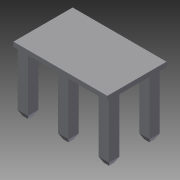
# Autodesk Inventor part: TMM-103-05-F-D_pins2
Saved by Autodesk Inventor 2014 SP2 (Build 180246200, 246)
## iProperties
Created: 2019-03-13
Part Number: TMM-103-05-F-D_pins2
Material: Generic
Catalog Web Link: www.cadenas.de
Description: TMM pins2-TMM Series
Vendor: SAMTEC
Document SubType Name: Modeling
Designer: psadmin
Manufacturer: SAMTEC
Mass: 0.00765058 g
Surface Area: 0.660321 cm^2
Volume: 0.00765058 cm^3
Density: 1 g/cm^3
Appearance: PSOLRGB-191-191-191
Category: PARTsolutions
Company: SAMTEC
Title: TMM-103-05-F-D_pins2
Author: Cadenas PARTsolutions
Comments: TMM Series
PSOL_IDENT_0: {$CADENAS_DATA\23d-libs\samtec\modelling\tmm\parts\tmm_pins2.prj},233 {VTYP=3D},{NB=TMM-103-05-F-D_p
PSOL_IDENT_1: ins2},{LINA=TMM-103-05-F-D_pins2},{NN=TMM pins2},{DATE=15.05.2015 12:28:13},{GEOMDATE=13.11.2014 09:
PSOL_IDENT_2: 06:00},{VERSION=},{LINEID=10},{WBVAR=POS,LS,PLOPT,ROW,TOPT,AOPT,RCOPT,POLOPT,KOPT,TROPT},{WBNUMERIC=
PSOL_IDENT_3: }  {NB=TMM-103-05-F-D_pins2},{LINA=TMM-103-05-F-D_pins2},{KT=DUMMY},{PN=TMM-103-05-F-D},{SERIES=TMM}
PSOL_IDENT_4: ,{POS=03},{LS=05},{LEADSTALG=},{PLOPT=F},{PLOPTALG= '-L','10micro\" (0,25 microm) Gold on contact, M
PSOL_IDENT_5: atte Tin on tail','-S','30micro\" (0,76 microm) Gold on contact, Matte Tin on tail' },{ROW=D},{ROWOP
PSOL_IDENT_6: TALG= 'S','S:Single row','D','D:Double Row','Q','Q:Quad Row' },{TOPT=},{TOPTALG= '','Straight','-SM'
PSOL_IDENT_7: ,'SM: Surface Mount' },{SH=160},{STACKERHALG=[120:323/5]},{TAILL=090},{TAILLALG='000','005','010','0
PSOL_IDENT_8: 15','020','025','030','035','040','045','050','055','060','065','070','075','080','085','090','095','
PSOL_IDENT_9: 100','105','110','115','120','125','130','135','140','145','150','155','160'},{AOPT=},{AOPTALG= '','
PSOL_IDENT_10: Not Available' },{RCOPT=},{RCOPTALG= '','Not Available' },{POLOPT=Not Selected},{POLARIZEALG='001','
PSOL_IDENT_11: 002','003','004','005','006'},{POLARIZEPN=},{KOPT=},{KOPTALG= '','Not Available' },{TROPT=},{TROPTAL
PSOL_IDENT_12: G= '','Not Available' },{L=0.23622},{W=0.1574},{OAL=0.323},{STACKERHMAX=323},{POLMAX='001','002','00
PSOL_IDENT_13: 3','004','005','006','007','008','009','010','011','012','013','014','015','016','017','018','019','
PSOL_IDENT_14: 020','021','022','023','024','025','026','027','028','029','030','031','032','033','034','035','036'
PSOL_IDENT_15: ,'037','038','039','040','041','042','043','044','045','046','047','048','049','050','051','052','05
PSOL_IDENT_16: 3','054','055','056','057','058','059','060','061','062','063','064','065','066','067','068','069','
PSOL_IDENT_17: 070','071','072','073','074','075','076','077','078','079','080','081','082','083','084','085','086'
PSOL_IDENT_18: ,'087','088','089','090','091','092','093','094','095','096','097','098','099','100','101','102','10
PSOL_IDENT_19: 3','104','105','106','107','108','109','110','111','112','113','114','115','116','117','118','119','
PSOL_IDENT_20: 120','121','122','123','124','125','126','127','128','129','130','131','132','133','134','135','136'
PSOL_IDENT_21: ,'137','138','139','140','141','142','143','144','145','146','147','148','149','150','151','152','15
PSOL_IDENT_22: 3','154','155','156','157','158','159','160','161','162','163','164','165','166','167','168','169','
PSOL_IDENT_23: 170','171','172','173','174','175','176','177','178','179','180','181','182','183','184','185','186'
PSOL_IDENT_24: ,'187','188','189','190','191','192','193','194','195','196','197','198','199','200','201','202','20
PSOL_IDENT_25: 3','204','205','206','207','208','209','210','211','212','213','214','215','216','217','218','219','
PSOL_IDENT_26: 220','221','222','223','224','225','226','227','228','229','230','231','232','233','234','235','236'
PSOL_IDENT_27: ,'237','238','239','240','241','242','243','244','245','246','247','248','249','250','251','252','25
PSOL_IDENT_28: 3','254','255','256','257','258','259','260','261','262','263','264','265','266','267','268','269','
PSOL_IDENT_29: 270','271','272','273','274','275','276','277','278','279','280','281','282','283','284','285','286'
PSOL_IDENT_30: ,'287','288','289','290','291','292','293','294','295','296','297','298','299','300'},{TEST2='001','
PSOL_IDENT_31: 002','003','004','005','006'},{TRUNC=6},{MIN=0.163},{PINSNUM=3},{POLLR=0},{TAILLMAX=163},{TAILLRANGE='
PSOL_IDENT_32: 000','005','010','015','020','025','030','035','040','045','050','055','060','065','070','075','080'
PSOL_IDENT_33: ,'085','090','095','100','105','110','115','120','125','130','135','140','145','150','155','160','16
PSOL_IDENT_34: 5','170','175','180','185','190','195','200','205','210','215','220','225','230','235','240','245','
PSOL_IDENT_35: 250','255','260','265','270','275','280','285','290','295','300','305','310','315','320','325','330'
PSOL_IDENT_36: ,'335','340','345','350','355','360','365','370','375','380','385','390','395','400','405','410','41
PSOL_IDENT_37: 5','420','425','430','435','440','445','450','455','460','465','470','475','480','485','490','495','
PSOL_IDENT_38: 500','505','510','515','520','525','530','535','540','545','550','555','560','565','570','575','580'
PSOL_IDENT_39: ,'585','590','595','600','605','610','615','620','625','630','635','640','645','650','655','660','66
PSOL_IDENT_40: 5','670','675','680','685','690','695','700','705','710','715','720','725','730','735','740','745','
PSOL_IDENT_41: 750','755','760','765','770','775','780','785','790','795','800','805','810','815','820','825','830'
PSOL_IDENT_42: ,'835','840','845','850','855','860','865','870','875','880','885','890','895','900','905','910','91
PSOL_IDENT_43: 5','920','925','930','935','940','945','950','955','960','965','970','975','980','985','990','995'},
PSOL_IDENT_44: {TAILLTRUNC=33},{TAILLNUM=0.09},{ROWNO=2},{POLPLANEPOS=0},{POLPINPOS=0},{TOPCUT=0.198},{COLOR=0.75,0
PSOL_IDENT_45: .75,0.75,0.00}
NN: TMM pins2
NT: TMM Series
NB: TMM-103-05-F-D_pins2
NBSYN: $PN._pins2
LINA: TMM-103-05-F-D_pins2
SERIES: TMM
POS: 03
LS: 05
PLOPT: -F: 3u" Selective Gold on Contact, Matte Tin on Tail
ROW: D:Double Row
TOPT: Straight
SH: 160
AOPT: Not Available
RCOPT: Not Available
POLOPT: Not Selected
KOPT: Not Available
TROPT: Not Available
POLMAX: '001','002','003','004','005','006','007','008','009','010','011','012','013','014','015','016','017','018','019','020','021','022','023','024','025','026','027','028','029','030','031','032','033','034','035','036','037','038','039','040','041','042','043','044','045','046','047','048','049','050','051','052','053','054','055','056','057','058','059','060','061','062','063','064','065','066','067','068','069','070','071','072','073','074','075','076','077','078','079','080','081','082','083','084','085','086','087','088','089','090','091','092','093','094','095','096','097','098','099','100','101','102','103','104','105','106','107','108','109','110','111','112','113','114','115','116','117','118','119','120','121','122','123','124','125','126','127','128','129','130','131','132','133','134','135','136','137','138','139','140','141','142','143','144','145','146','147','148','149','150','151','152','153','154','155','156','157','158','159','160','161','162','163','164','165','166','167','168','169','170','171','172','173','174','175','176','177','178','179','180','181','182','183','184','185','186','187','188','189','190','191','192','193','194','195','196','197','198','199','200','201','202','203','204','205','206','207','208','209','210','211','212','213','214','215','216','217','218','219','220','221','222','223','224','225','226','227','228','229','230','231','232','233','234','235','236','237','238','239','240','241','242','243','244','245','246','247','248','249','250','251','252','253','254','255','256','257','258','259','260','261','262','263','264','265','266','267','268','269','270','271','272','273','274','275','276','277','278','279','280','281','282','283','284','285','286','287','288','289','290','291','292','293','294','295','296','297','298','299','300'
TAILLRANGE: '000','005','010','015','020','025','030','035','040','045','050','055','060','065','070','075','080','085','090','095','100','105','110','115','120','125','130','135','140','145','150','155','160','165','170','175','180','185','190','195','200','205','210','215','220','225','230','235','240','245','250','255','260','265','270','275','280','285','290','295','300','305','310','315','320','325','330','335','340','345','350','355','360','365','370','375','380','385','390','395','400','405','410','415','420','425','430','435','440','445','450','455','460','465','470','475','480','485','490','495','500','505','510','515','520','525','530','535','540','545','550','555','560','565','570','575','580','585','590','595','600','605','610','615','620','625','630','635','640','645','650','655','660','665','670','675','680','685','690','695','700','705','710','715','720','725','730','735','740','745','750','755','760','765','770','775','780','785','790','795','800','805','810','815','820','825','830','835','840','845','850','855','860','865','870','875','880','885','890','895','900','905','910','915','920','925','930','935','940','945','950','955','960','965','970','975','980','985','990','995'
SUPPLIER: SAMTEC
ARTICLENO: TMM-103-05-F-D_pins2
BOMINFO: TMM-103-05-F-D_pins2
CREATOR: CADENAS GmbH
Autodesk Inventor part; units mm, degrees
ref_plane "YZ Plane" through (0, 0, 0) normal (1, 0, 0) x (0, 1, 0)
ref_plane "XZ Plane" through (0, 0, 0) normal (0, 1, 0) x (-1, 0, 0)
ref_plane "XY Plane" through (0, 0, 0) normal (0, 0, 1) x (1, 0, 0)
sketch "Sketch_2" plane through (-2.254, 0, 0) normal (1, 0, 0) x (0, 0, -1)
  line L0 (-1.4605, 0.762) -> (-1.254, 0.762)
  line L1 (-1.254, 0.762) -> (-1.254, -2.032)
  line L2 (-1.254, -2.032) -> (-1.127, -2.286)
  line L3 (-1.127, -2.286) -> (-0.873, -2.286)
  line L4 (-0.873, -2.286) -> (-0.746, -2.032)
  line L5 (-0.746, -2.032) -> (-0.746, 0.762)
  line L6 (-0.746, 0.762) -> (0.746, 0.762)
  line L7 (0.746, 0.762) -> (0.746, -2.032)
  line L8 (0.746, -2.032) -> (0.873, -2.286)
  line L9 (0.873, -2.286) -> (1.127, -2.286)
  line L10 (1.127, -2.286) -> (1.254, -2.032)
  line L11 (1.254, -2.032) -> (1.254, 0.762)
  line L12 (1.254, 0.762) -> (1.4605, 0.762)
  line L13 (1.4605, 0.762) -> (1.4605, 0.9906)
  line L14 (1.4605, 0.9906) -> (-1.4605, 0.9906)
  line L15 (-1.4605, 0.9906) -> (-1.4605, 0.762)
  constraints: 32 end point
extrude "Extrusion1" add sketch "Sketch_2" along normal blind 4.635
sketch "Sketch_1" plane through (0, 0, 0) normal (0, 0, 1) x (1, 0, 0)
  line L0 (-109.4334, 38.1) -> (-109.4334, -38.1)
  line L1 (-109.4334, -38.1) -> (56.7986, -38.1)
  line L2 (56.7986, -38.1) -> (56.7986, 38.1)
  line L3 (56.7986, 38.1) -> (-109.4334, 38.1)
  line L4 (-100.4603, 0.762) -> (-100.2538, 0.762)
  line L5 (-100.2538, 0.762) -> (-100.2538, -2.032)
  line L6 (-100.2538, -2.032) -> (-100.1268, -2.286)
  line L7 (-100.1268, -2.286) -> (-99.8728, -2.286)
  line L8 (-99.8728, -2.286) -> (-99.7458, -2.032)
  line L9 (-99.7458, -2.032) -> (-99.7458, 0.762)
  line L10 (-99.7458, 0.762) -> (-98.2538, 0.762)
  line L11 (-98.2538, 0.762) -> (-98.2538, -2.032)
  line L12 (-98.2538, -2.032) -> (-98.1268, -2.286)
  line L13 (-98.1268, -2.286) -> (-97.8728, -2.286)
  line L14 (-97.8728, -2.286) -> (-97.7458, -2.032)
  line L15 (-97.7458, -2.032) -> (-97.7458, 0.762)
  line L16 (-97.7458, 0.762) -> (-96.2538, 0.762)
  line L17 (-96.2538, 0.762) -> (-96.2538, -2.032)
  line L18 (-96.2538, -2.032) -> (-96.1268, -2.286)
  line L19 (-96.1268, -2.286) -> (-95.8728, -2.286)
  line L20 (-95.8728, -2.286) -> (-95.7458, -2.032)
  line L21 (-95.7458, -2.032) -> (-95.7458, 0.762)
  line L22 (-95.7458, 0.762) -> (-94.2538, 0.762)
  line L23 (-94.2538, 0.762) -> (-94.2538, -2.032)
  line L24 (-94.2538, -2.032) -> (-94.1268, -2.286)
  line L25 (-94.1268, -2.286) -> (-93.8728, -2.286)
  line L26 (-93.8728, -2.286) -> (-93.7458, -2.032)
  line L27 (-93.7458, -2.032) -> (-93.7458, 0.762)
  line L28 (-93.7458, 0.762) -> (-92.2538, 0.762)
  line L29 (-92.2538, 0.762) -> (-92.2538, -2.032)
  line L30 (-92.2538, -2.032) -> (-92.1268, -2.286)
  line L31 (-92.1268, -2.286) -> (-91.8728, -2.286)
  line L32 (-91.8728, -2.286) -> (-91.7458, -2.032)
  line L33 (-91.7458, -2.032) -> (-91.7458, 0.762)
  line L34 (-91.7458, 0.762) -> (-90.2538, 0.762)
  line L35 (-90.2538, 0.762) -> (-90.2538, -2.032)
  line L36 (-90.2538, -2.032) -> (-90.1268, -2.286)
  line L37 (-90.1268, -2.286) -> (-89.8728, -2.286)
  line L38 (-89.8728, -2.286) -> (-89.7458, -2.032)
  line L39 (-89.7458, -2.032) -> (-89.7458, 0.762)
  line L40 (-89.7458, 0.762) -> (-88.2538, 0.762)
  line L41 (-88.2538, 0.762) -> (-88.2538, -2.032)
  line L42 (-88.2538, -2.032) -> (-88.1268, -2.286)
  line L43 (-88.1268, -2.286) -> (-87.8728, -2.286)
  line L44 (-87.8728, -2.286) -> (-87.7458, -2.032)
  line L45 (-87.7458, -2.032) -> (-87.7458, 0.762)
  line L46 (-87.7458, 0.762) -> (-86.2538, 0.762)
  line L47 (-86.2538, 0.762) -> (-86.2538, -2.032)
  line L48 (-86.2538, -2.032) -> (-86.1268, -2.286)
  line L49 (-86.1268, -2.286) -> (-85.8728, -2.286)
  line L50 (-85.8728, -2.286) -> (-85.7458, -2.032)
  line L51 (-85.7458, -2.032) -> (-85.7458, 0.762)
  line L52 (-85.7458, 0.762) -> (-84.2538, 0.762)
  line L53 (-84.2538, 0.762) -> (-84.2538, -2.032)
  line L54 (-84.2538, -2.032) -> (-84.1268, -2.286)
  line L55 (-84.1268, -2.286) -> (-83.8728, -2.286)
  line L56 (-83.8728, -2.286) -> (-83.7458, -2.032)
  line L57 (-83.7458, -2.032) -> (-83.7458, 0.762)
  line L58 (-83.7458, 0.762) -> (-82.2538, 0.762)
  line L59 (-82.2538, 0.762) -> (-82.2538, -2.032)
  line L60 (-82.2538, -2.032) -> (-82.1268, -2.286)
  line L61 (-82.1268, -2.286) -> (-81.8728, -2.286)
  line L62 (-81.8728, -2.286) -> (-81.7458, -2.032)
  line L63 (-81.7458, -2.032) -> (-81.7458, 0.762)
  line L64 (-81.7458, 0.762) -> (-80.2538, 0.762)
  line L65 (-80.2538, 0.762) -> (-80.2538, -2.032)
  line L66 (-80.2538, -2.032) -> (-80.1268, -2.286)
  line L67 (-80.1268, -2.286) -> (-79.8728, -2.286)
  line L68 (-79.8728, -2.286) -> (-79.7458, -2.032)
  line L69 (-79.7458, -2.032) -> (-79.7458, 0.762)
  line L70 (-79.7458, 0.762) -> (-78.2538, 0.762)
  line L71 (-78.2538, 0.762) -> (-78.2538, -2.032)
  line L72 (-78.2538, -2.032) -> (-78.1268, -2.286)
  line L73 (-78.1268, -2.286) -> (-77.8728, -2.286)
  line L74 (-77.8728, -2.286) -> (-77.7458, -2.032)
  line L75 (-77.7458, -2.032) -> (-77.7458, 0.762)
  line L76 (-77.7458, 0.762) -> (-76.2538, 0.762)
  line L77 (-76.2538, 0.762) -> (-76.2538, -2.032)
  line L78 (-76.2538, -2.032) -> (-76.1268, -2.286)
  line L79 (-76.1268, -2.286) -> (-75.8728, -2.286)
  line L80 (-75.8728, -2.286) -> (-75.7458, -2.032)
  line L81 (-75.7458, -2.032) -> (-75.7458, 0.762)
  line L82 (-75.7458, 0.762) -> (-74.2539, 0.762)
  line L83 (-74.2539, 0.762) -> (-74.2539, -2.032)
  line L84 (-74.2539, -2.032) -> (-74.1269, -2.286)
  line L85 (-74.1269, -2.286) -> (-73.8729, -2.286)
  line L86 (-73.8729, -2.286) -> (-73.7459, -2.032)
  line L87 (-73.7459, -2.032) -> (-73.7459, 0.762)
  line L88 (-73.7459, 0.762) -> (-72.2539, 0.762)
  line L89 (-72.2539, 0.762) -> (-72.2539, -2.032)
  line L90 (-72.2539, -2.032) -> (-72.1269, -2.286)
  line L91 (-72.1269, -2.286) -> (-71.8729, -2.286)
  line L92 (-71.8729, -2.286) -> (-71.7459, -2.032)
  line L93 (-71.7459, -2.032) -> (-71.7459, 0.762)
  line L94 (-71.7459, 0.762) -> (-70.2539, 0.762)
  line L95 (-70.2539, 0.762) -> (-70.2539, -2.032)
  line L96 (-70.2539, -2.032) -> (-70.1269, -2.286)
  line L97 (-70.1269, -2.286) -> (-69.8729, -2.286)
  line L98 (-69.8729, -2.286) -> (-69.7459, -2.032)
  line L99 (-69.7459, -2.032) -> (-69.7459, 0.762)
  line L100 (-69.7459, 0.762) -> (-68.2539, 0.762)
  line L101 (-68.2539, 0.762) -> (-68.2539, -2.032)
  line L102 (-68.2539, -2.032) -> (-68.1269, -2.286)
  line L103 (-68.1269, -2.286) -> (-67.8729, -2.286)
  line L104 (-67.8729, -2.286) -> (-67.7459, -2.032)
  line L105 (-67.7459, -2.032) -> (-67.7459, 0.762)
  line L106 (-67.7459, 0.762) -> (-66.2539, 0.762)
  line L107 (-66.2539, 0.762) -> (-66.2539, -2.032)
  line L108 (-66.2539, -2.032) -> (-66.1269, -2.286)
  line L109 (-66.1269, -2.286) -> (-65.8729, -2.286)
  line L110 (-65.8729, -2.286) -> (-65.7459, -2.032)
  line L111 (-65.7459, -2.032) -> (-65.7459, 0.762)
  line L112 (-65.7459, 0.762) -> (-64.2539, 0.762)
  line L113 (-64.2539, 0.762) -> (-64.2539, -2.032)
  line L114 (-64.2539, -2.032) -> (-64.1269, -2.286)
  line L115 (-64.1269, -2.286) -> (-63.8729, -2.286)
  line L116 (-63.8729, -2.286) -> (-63.7459, -2.032)
  line L117 (-63.7459, -2.032) -> (-63.7459, 0.762)
  line L118 (-63.7459, 0.762) -> (-62.2539, 0.762)
  line L119 (-62.2539, 0.762) -> (-62.2539, -2.032)
  line L120 (-62.2539, -2.032) -> (-62.1269, -2.286)
  line L121 (-62.1269, -2.286) -> (-61.8729, -2.286)
  line L122 (-61.8729, -2.286) -> (-61.7459, -2.032)
  line L123 (-61.7459, -2.032) -> (-61.7459, 0.762)
  line L124 (-61.7459, 0.762) -> (-60.2539, 0.762)
  line L125 (-60.2539, 0.762) -> (-60.2539, -2.032)
  line L126 (-60.2539, -2.032) -> (-60.1269, -2.286)
  line L127 (-60.1269, -2.286) -> (-59.8729, -2.286)
  line L128 (-59.8729, -2.286) -> (-59.7459, -2.032)
  line L129 (-59.7459, -2.032) -> (-59.7459, 0.762)
  line L130 (-59.7459, 0.762) -> (-58.2539, 0.762)
  line L131 (-58.2539, 0.762) -> (-58.2539, -2.032)
  line L132 (-58.2539, -2.032) -> (-58.1269, -2.286)
  line L133 (-58.1269, -2.286) -> (-57.8729, -2.286)
  line L134 (-57.8729, -2.286) -> (-57.7459, -2.032)
  line L135 (-57.7459, -2.032) -> (-57.7459, 0.762)
  line L136 (-57.7459, 0.762) -> (-56.2539, 0.762)
  line L137 (-56.2539, 0.762) -> (-56.2539, -2.032)
  line L138 (-56.2539, -2.032) -> (-56.1269, -2.286)
  line L139 (-56.1269, -2.286) -> (-55.8729, -2.286)
  line L140 (-55.8729, -2.286) -> (-55.7459, -2.032)
  line L141 (-55.7459, -2.032) -> (-55.7459, 0.762)
  line L142 (-55.7459, 0.762) -> (-54.2539, 0.762)
  line L143 (-54.2539, 0.762) -> (-54.2539, -2.032)
  line L144 (-54.2539, -2.032) -> (-54.1269, -2.286)
  line L145 (-54.1269, -2.286) -> (-53.8729, -2.286)
  line L146 (-53.8729, -2.286) -> (-53.7459, -2.032)
  line L147 (-53.7459, -2.032) -> (-53.7459, 0.762)
  line L148 (-53.7459, 0.762) -> (-52.2539, 0.762)
  line L149 (-52.2539, 0.762) -> (-52.2539, -2.032)
  line L150 (-52.2539, -2.032) -> (-52.1269, -2.286)
  line L151 (-52.1269, -2.286) -> (-51.8729, -2.286)
  line L152 (-51.8729, -2.286) -> (-51.7459, -2.032)
  line L153 (-51.7459, -2.032) -> (-51.7459, 0.762)
  line L154 (-51.7459, 0.762) -> (-50.2539, 0.762)
  line L155 (-50.2539, 0.762) -> (-50.2539, -2.032)
  line L156 (-50.2539, -2.032) -> (-50.1269, -2.286)
  line L157 (-50.1269, -2.286) -> (-49.8729, -2.286)
  line L158 (-49.8729, -2.286) -> (-49.7459, -2.032)
  line L159 (-49.7459, -2.032) -> (-49.7459, 0.762)
  line L160 (-49.7459, 0.762) -> (-48.2539, 0.762)
  line L161 (-48.2539, 0.762) -> (-48.2539, -2.032)
  line L162 (-48.2539, -2.032) -> (-48.1269, -2.286)
  line L163 (-48.1269, -2.286) -> (-47.8729, -2.286)
  line L164 (-47.8729, -2.286) -> (-47.7459, -2.032)
  line L165 (-47.7459, -2.032) -> (-47.7459, 0.762)
  line L166 (-47.7459, 0.762) -> (-46.2539, 0.762)
  line L167 (-46.2539, 0.762) -> (-46.2539, -2.032)
  line L168 (-46.2539, -2.032) -> (-46.1269, -2.286)
  line L169 (-46.1269, -2.286) -> (-45.8729, -2.286)
  line L170 (-45.8729, -2.286) -> (-45.7459, -2.032)
  line L171 (-45.7459, -2.032) -> (-45.7459, 0.762)
  line L172 (-45.7459, 0.762) -> (-44.2539, 0.762)
  line L173 (-44.2539, 0.762) -> (-44.2539, -2.032)
  line L174 (-44.2539, -2.032) -> (-44.1269, -2.286)
  line L175 (-44.1269, -2.286) -> (-43.8729, -2.286)
  line L176 (-43.8729, -2.286) -> (-43.7459, -2.032)
  line L177 (-43.7459, -2.032) -> (-43.7459, 0.762)
  line L178 (-43.7459, 0.762) -> (-42.2539, 0.762)
  line L179 (-42.2539, 0.762) -> (-42.2539, -2.032)
  line L180 (-42.2539, -2.032) -> (-42.1269, -2.286)
  line L181 (-42.1269, -2.286) -> (-41.8729, -2.286)
  line L182 (-41.8729, -2.286) -> (-41.7459, -2.032)
  line L183 (-41.7459, -2.032) -> (-41.7459, 0.762)
  line L184 (-41.7459, 0.762) -> (-40.2539, 0.762)
  line L185 (-40.2539, 0.762) -> (-40.2539, -2.032)
  line L186 (-40.2539, -2.032) -> (-40.1269, -2.286)
  line L187 (-40.1269, -2.286) -> (-39.8729, -2.286)
  line L188 (-39.8729, -2.286) -> (-39.7459, -2.032)
  line L189 (-39.7459, -2.032) -> (-39.7459, 0.762)
  line L190 (-39.7459, 0.762) -> (-38.2539, 0.762)
  line L191 (-38.2539, 0.762) -> (-38.2539, -2.032)
  line L192 (-38.2539, -2.032) -> (-38.1269, -2.286)
  line L193 (-38.1269, -2.286) -> (-37.8729, -2.286)
  line L194 (-37.8729, -2.286) -> (-37.7459, -2.032)
  line L195 (-37.7459, -2.032) -> (-37.7459, 0.762)
  line L196 (-37.7459, 0.762) -> (-36.2539, 0.762)
  line L197 (-36.2539, 0.762) -> (-36.2539, -2.032)
  line L198 (-36.2539, -2.032) -> (-36.1269, -2.286)
  line L199 (-36.1269, -2.286) -> (-35.8729, -2.286)
  line L200 (-35.8729, -2.286) -> (-35.7459, -2.032)
  line L201 (-35.7459, -2.032) -> (-35.7459, 0.762)
  line L202 (-35.7459, 0.762) -> (-34.2539, 0.762)
  line L203 (-34.2539, 0.762) -> (-34.2539, -2.032)
  line L204 (-34.2539, -2.032) -> (-34.1269, -2.286)
  line L205 (-34.1269, -2.286) -> (-33.8729, -2.286)
  line L206 (-33.8729, -2.286) -> (-33.7459, -2.032)
  line L207 (-33.7459, -2.032) -> (-33.7459, 0.762)
  line L208 (-33.7459, 0.762) -> (-32.2539, 0.762)
  line L209 (-32.2539, 0.762) -> (-32.2539, -2.032)
  line L210 (-32.2539, -2.032) -> (-32.1269, -2.286)
  line L211 (-32.1269, -2.286) -> (-31.8729, -2.286)
  line L212 (-31.8729, -2.286) -> (-31.7459, -2.032)
  line L213 (-31.7459, -2.032) -> (-31.7459, 0.762)
  line L214 (-31.7459, 0.762) -> (-30.2539, 0.762)
  line L215 (-30.2539, 0.762) -> (-30.2539, -2.032)
  line L216 (-30.2539, -2.032) -> (-30.1269, -2.286)
  line L217 (-30.1269, -2.286) -> (-29.8729, -2.286)
  line L218 (-29.8729, -2.286) -> (-29.7459, -2.032)
  line L219 (-29.7459, -2.032) -> (-29.7459, 0.762)
  line L220 (-29.7459, 0.762) -> (-28.2539, 0.762)
  line L221 (-28.2539, 0.762) -> (-28.2539, -2.032)
  line L222 (-28.2539, -2.032) -> (-28.1269, -2.286)
  line L223 (-28.1269, -2.286) -> (-27.8729, -2.286)
  line L224 (-27.8729, -2.286) -> (-27.7459, -2.032)
  line L225 (-27.7459, -2.032) -> (-27.7459, 0.762)
  line L226 (-27.7459, 0.762) -> (-26.2539, 0.762)
  line L227 (-26.2539, 0.762) -> (-26.2539, -2.032)
  line L228 (-26.2539, -2.032) -> (-26.1269, -2.286)
  line L229 (-26.1269, -2.286) -> (-25.8729, -2.286)
  line L230 (-25.8729, -2.286) -> (-25.7459, -2.032)
  line L231 (-25.7459, -2.032) -> (-25.7459, 0.762)
  line L232 (-25.7459, 0.762) -> (-24.254, 0.762)
  line L233 (-24.254, 0.762) -> (-24.254, -2.032)
  line L234 (-24.254, -2.032) -> (-24.127, -2.286)
  line L235 (-24.127, -2.286) -> (-23.873, -2.286)
  line L236 (-23.873, -2.286) -> (-23.746, -2.032)
  line L237 (-23.746, -2.032) -> (-23.746, 0.762)
  line L238 (-23.746, 0.762) -> (-22.254, 0.762)
  line L239 (-22.254, 0.762) -> (-22.254, -2.032)
  line L240 (-22.254, -2.032) -> (-22.127, -2.286)
  line L241 (-22.127, -2.286) -> (-21.873, -2.286)
  line L242 (-21.873, -2.286) -> (-21.746, -2.032)
  line L243 (-21.746, -2.032) -> (-21.746, 0.762)
  line L244 (-21.746, 0.762) -> (-20.254, 0.762)
  line L245 (-20.254, 0.762) -> (-20.254, -2.032)
  line L246 (-20.254, -2.032) -> (-20.127, -2.286)
  line L247 (-20.127, -2.286) -> (-19.873, -2.286)
  line L248 (-19.873, -2.286) -> (-19.746, -2.032)
  line L249 (-19.746, -2.032) -> (-19.746, 0.762)
  line L250 (-19.746, 0.762) -> (-18.254, 0.762)
  line L251 (-18.254, 0.762) -> (-18.254, -2.032)
  line L252 (-18.254, -2.032) -> (-18.127, -2.286)
  line L253 (-18.127, -2.286) -> (-17.873, -2.286)
  line L254 (-17.873, -2.286) -> (-17.746, -2.032)
  line L255 (-17.746, -2.032) -> (-17.746, 0.762)
  line L256 (-17.746, 0.762) -> (-16.254, 0.762)
  line L257 (-16.254, 0.762) -> (-16.254, -2.032)
  line L258 (-16.254, -2.032) -> (-16.127, -2.286)
  line L259 (-16.127, -2.286) -> (-15.873, -2.286)
  line L260 (-15.873, -2.286) -> (-15.746, -2.032)
  line L261 (-15.746, -2.032) -> (-15.746, 0.762)
  line L262 (-15.746, 0.762) -> (-14.254, 0.762)
  line L263 (-14.254, 0.762) -> (-14.254, -2.032)
  line L264 (-14.254, -2.032) -> (-14.127, -2.286)
  line L265 (-14.127, -2.286) -> (-13.873, -2.286)
  line L266 (-13.873, -2.286) -> (-13.746, -2.032)
  line L267 (-13.746, -2.032) -> (-13.746, 0.762)
  line L268 (-13.746, 0.762) -> (-12.254, 0.762)
  line L269 (-12.254, 0.762) -> (-12.254, -2.032)
  line L270 (-12.254, -2.032) -> (-12.127, -2.286)
  line L271 (-12.127, -2.286) -> (-11.873, -2.286)
  line L272 (-11.873, -2.286) -> (-11.746, -2.032)
  line L273 (-11.746, -2.032) -> (-11.746, 0.762)
  line L274 (-11.746, 0.762) -> (-10.254, 0.762)
  line L275 (-10.254, 0.762) -> (-10.254, -2.032)
  line L276 (-10.254, -2.032) -> (-10.127, -2.286)
  line L277 (-10.127, -2.286) -> (-9.873, -2.286)
  line L278 (-9.873, -2.286) -> (-9.746, -2.032)
  line L279 (-9.746, -2.032) -> (-9.746, 0.762)
  line L280 (-9.746, 0.762) -> (-8.254, 0.762)
  line L281 (-8.254, 0.762) -> (-8.254, -2.032)
  line L282 (-8.254, -2.032) -> (-8.127, -2.286)
  line L283 (-8.127, -2.286) -> (-7.873, -2.286)
  line L284 (-7.873, -2.286) -> (-7.746, -2.032)
  line L285 (-7.746, -2.032) -> (-7.746, 0.762)
  line L286 (-7.746, 0.762) -> (-6.254, 0.762)
  line L287 (-6.254, 0.762) -> (-6.254, -2.032)
  line L288 (-6.254, -2.032) -> (-6.127, -2.286)
  line L289 (-6.127, -2.286) -> (-5.873, -2.286)
  line L290 (-5.873, -2.286) -> (-5.746, -2.032)
  line L291 (-5.746, -2.032) -> (-5.746, 0.762)
  line L292 (-5.746, 0.762) -> (-4.254, 0.762)
  line L293 (-4.254, 0.762) -> (-4.254, -2.032)
  line L294 (-4.254, -2.032) -> (-4.127, -2.286)
  line L295 (-4.127, -2.286) -> (-3.873, -2.286)
  line L296 (-3.873, -2.286) -> (-3.746, -2.032)
  line L297 (-3.746, -2.032) -> (-3.746, 0.762)
  line L298 (-3.746, 0.762) -> (-2.254, 0.762)
  line L299 (-2.254, 0.762) -> (-2.254, -2.032)
  line L300 (-2.254, -2.032) -> (-2.127, -2.286)
  line L301 (-2.127, -2.286) -> (-1.873, -2.286)
  line L302 (-1.873, -2.286) -> (-1.746, -2.032)
  line L303 (-1.746, -2.032) -> (-1.746, 0.762)
  line L304 (-1.746, 0.762) -> (-0.254, 0.762)
  line L305 (-0.254, 0.762) -> (-0.254, -2.032)
  line L306 (-0.254, -2.032) -> (-0.127, -2.286)
  line L307 (-0.127, -2.286) -> (0.127, -2.286)
  line L308 (0.127, -2.286) -> (0.254, -2.032)
  line L309 (0.254, -2.032) -> (0.254, 0.762)
  line L310 (0.254, 0.762) -> (1.746, 0.762)
  line L311 (1.746, 0.762) -> (1.746, -2.032)
  line L312 (1.746, -2.032) -> (1.873, -2.286)
  line L313 (1.873, -2.286) -> (2.127, -2.286)
  line L314 (2.127, -2.286) -> (2.254, -2.032)
  line L315 (2.254, -2.032) -> (2.254, 0.762)
  line L316 (2.254, 0.762) -> (2.4605, 0.762)
  line L317 (2.4605, 0.762) -> (2.4605, 0.9906)
  line L318 (2.4605, 0.9906) -> (2.254, 0.9906)
  line L319 (2.254, 0.9906) -> (2.254, 5.6642)
  line L320 (2.254, 5.6642) -> (2.127, 5.9182)
  line L321 (2.127, 5.9182) -> (1.873, 5.9182)
  line L322 (1.873, 5.9182) -> (1.746, 5.6642)
  line L323 (1.746, 5.6642) -> (1.746, 0.9906)
  line L324 (1.746, 0.9906) -> (0.254, 0.9906)
  line L325 (0.254, 0.9906) -> (0.254, 5.6642)
  line L326 (0.254, 5.6642) -> (0.127, 5.9182)
  line L327 (0.127, 5.9182) -> (-0.127, 5.9182)
  line L328 (-0.127, 5.9182) -> (-0.254, 5.6642)
  line L329 (-0.254, 5.6642) -> (-0.254, 0.9906)
  line L330 (-0.254, 0.9906) -> (-1.746, 0.9906)
  line L331 (-1.746, 0.9906) -> (-1.746, 5.6642)
  line L332 (-1.746, 5.6642) -> (-1.873, 5.9182)
  line L333 (-1.873, 5.9182) -> (-2.127, 5.9182)
  line L334 (-2.127, 5.9182) -> (-2.254, 5.6642)
  line L335 (-2.254, 5.6642) -> (-2.254, 0.9906)
  line L336 (-2.254, 0.9906) -> (-3.746, 0.9906)
  line L337 (-3.746, 0.9906) -> (-3.746, 5.6642)
  line L338 (-3.746, 5.6642) -> (-3.873, 5.9182)
  line L339 (-3.873, 5.9182) -> (-4.127, 5.9182)
  line L340 (-4.127, 5.9182) -> (-4.254, 5.6642)
  line L341 (-4.254, 5.6642) -> (-4.254, 0.9906)
  line L342 (-4.254, 0.9906) -> (-5.746, 0.9906)
  line L343 (-5.746, 0.9906) -> (-5.746, 5.6642)
  line L344 (-5.746, 5.6642) -> (-5.873, 5.9182)
  line L345 (-5.873, 5.9182) -> (-6.127, 5.9182)
  line L346 (-6.127, 5.9182) -> (-6.254, 5.6642)
  line L347 (-6.254, 5.6642) -> (-6.254, 0.9906)
  line L348 (-6.254, 0.9906) -> (-7.746, 0.9906)
  line L349 (-7.746, 0.9906) -> (-7.746, 5.6642)
  line L350 (-7.746, 5.6642) -> (-7.873, 5.9182)
  line L351 (-7.873, 5.9182) -> (-8.127, 5.9182)
  line L352 (-8.127, 5.9182) -> (-8.254, 5.6642)
  line L353 (-8.254, 5.6642) -> (-8.254, 0.9906)
  line L354 (-8.254, 0.9906) -> (-9.746, 0.9906)
  line L355 (-9.746, 0.9906) -> (-9.746, 5.6642)
  line L356 (-9.746, 5.6642) -> (-9.873, 5.9182)
  line L357 (-9.873, 5.9182) -> (-10.127, 5.9182)
  line L358 (-10.127, 5.9182) -> (-10.254, 5.6642)
  line L359 (-10.254, 5.6642) -> (-10.254, 0.9906)
  line L360 (-10.254, 0.9906) -> (-11.746, 0.9906)
  line L361 (-11.746, 0.9906) -> (-11.746, 5.6642)
  line L362 (-11.746, 5.6642) -> (-11.873, 5.9182)
  line L363 (-11.873, 5.9182) -> (-12.127, 5.9182)
  line L364 (-12.127, 5.9182) -> (-12.254, 5.6642)
  line L365 (-12.254, 5.6642) -> (-12.254, 0.9906)
  line L366 (-12.254, 0.9906) -> (-13.746, 0.9906)
  line L367 (-13.746, 0.9906) -> (-13.746, 5.6642)
  line L368 (-13.746, 5.6642) -> (-13.873, 5.9182)
  line L369 (-13.873, 5.9182) -> (-14.127, 5.9182)
  line L370 (-14.127, 5.9182) -> (-14.254, 5.6642)
  line L371 (-14.254, 5.6642) -> (-14.254, 0.9906)
  line L372 (-14.254, 0.9906) -> (-15.746, 0.9906)
  line L373 (-15.746, 0.9906) -> (-15.746, 5.6642)
  line L374 (-15.746, 5.6642) -> (-15.873, 5.9182)
  line L375 (-15.873, 5.9182) -> (-16.127, 5.9182)
  line L376 (-16.127, 5.9182) -> (-16.254, 5.6642)
  line L377 (-16.254, 5.6642) -> (-16.254, 0.9906)
  line L378 (-16.254, 0.9906) -> (-17.746, 0.9906)
  line L379 (-17.746, 0.9906) -> (-17.746, 5.6642)
  line L380 (-17.746, 5.6642) -> (-17.873, 5.9182)
  line L381 (-17.873, 5.9182) -> (-18.127, 5.9182)
  line L382 (-18.127, 5.9182) -> (-18.254, 5.6642)
  line L383 (-18.254, 5.6642) -> (-18.254, 0.9906)
  line L384 (-18.254, 0.9906) -> (-19.746, 0.9906)
  line L385 (-19.746, 0.9906) -> (-19.746, 5.6642)
  line L386 (-19.746, 5.6642) -> (-19.873, 5.9182)
  line L387 (-19.873, 5.9182) -> (-20.127, 5.9182)
  line L388 (-20.127, 5.9182) -> (-20.254, 5.6642)
  line L389 (-20.254, 5.6642) -> (-20.254, 0.9906)
  line L390 (-20.254, 0.9906) -> (-21.746, 0.9906)
  line L391 (-21.746, 0.9906) -> (-21.746, 5.6642)
  line L392 (-21.746, 5.6642) -> (-21.873, 5.9182)
  line L393 (-21.873, 5.9182) -> (-22.127, 5.9182)
  line L394 (-22.127, 5.9182) -> (-22.254, 5.6642)
  line L395 (-22.254, 5.6642) -> (-22.254, 0.9906)
  line L396 (-22.254, 0.9906) -> (-23.746, 0.9906)
  line L397 (-23.746, 0.9906) -> (-23.746, 5.6642)
  line L398 (-23.746, 5.6642) -> (-23.873, 5.9182)
  line L399 (-23.873, 5.9182) -> (-24.127, 5.9182)
  line L400 (-24.127, 5.9182) -> (-24.254, 5.6642)
  line L401 (-24.254, 5.6642) -> (-24.254, 0.9906)
  line L402 (-24.254, 0.9906) -> (-25.7459, 0.9906)
  line L403 (-25.7459, 0.9906) -> (-25.7459, 5.6642)
  line L404 (-25.7459, 5.6642) -> (-25.8729, 5.9182)
  line L405 (-25.8729, 5.9182) -> (-26.1269, 5.9182)
  line L406 (-26.1269, 5.9182) -> (-26.2539, 5.6642)
  line L407 (-26.2539, 5.6642) -> (-26.2539, 0.9906)
  line L408 (-26.2539, 0.9906) -> (-27.7459, 0.9906)
  line L409 (-27.7459, 0.9906) -> (-27.7459, 5.6642)
  line L410 (-27.7459, 5.6642) -> (-27.8729, 5.9182)
  line L411 (-27.8729, 5.9182) -> (-28.1269, 5.9182)
  line L412 (-28.1269, 5.9182) -> (-28.2539, 5.6642)
  line L413 (-28.2539, 5.6642) -> (-28.2539, 0.9906)
  line L414 (-28.2539, 0.9906) -> (-29.7459, 0.9906)
  line L415 (-29.7459, 0.9906) -> (-29.7459, 5.6642)
  line L416 (-29.7459, 5.6642) -> (-29.8729, 5.9182)
  line L417 (-29.8729, 5.9182) -> (-30.1269, 5.9182)
  line L418 (-30.1269, 5.9182) -> (-30.2539, 5.6642)
  line L419 (-30.2539, 5.6642) -> (-30.2539, 0.9906)
  line L420 (-30.2539, 0.9906) -> (-31.7459, 0.9906)
  line L421 (-31.7459, 0.9906) -> (-31.7459, 5.6642)
  line L422 (-31.7459, 5.6642) -> (-31.8729, 5.9182)
  line L423 (-31.8729, 5.9182) -> (-32.1269, 5.9182)
  line L424 (-32.1269, 5.9182) -> (-32.2539, 5.6642)
  line L425 (-32.2539, 5.6642) -> (-32.2539, 0.9906)
  line L426 (-32.2539, 0.9906) -> (-33.7459, 0.9906)
  line L427 (-33.7459, 0.9906) -> (-33.7459, 5.6642)
  line L428 (-33.7459, 5.6642) -> (-33.8729, 5.9182)
  line L429 (-33.8729, 5.9182) -> (-34.1269, 5.9182)
  line L430 (-34.1269, 5.9182) -> (-34.2539, 5.6642)
  line L431 (-34.2539, 5.6642) -> (-34.2539, 0.9906)
  line L432 (-34.2539, 0.9906) -> (-35.7459, 0.9906)
  line L433 (-35.7459, 0.9906) -> (-35.7459, 5.6642)
  line L434 (-35.7459, 5.6642) -> (-35.8729, 5.9182)
  line L435 (-35.8729, 5.9182) -> (-36.1269, 5.9182)
  line L436 (-36.1269, 5.9182) -> (-36.2539, 5.6642)
  line L437 (-36.2539, 5.6642) -> (-36.2539, 0.9906)
  line L438 (-36.2539, 0.9906) -> (-37.7459, 0.9906)
  line L439 (-37.7459, 0.9906) -> (-37.7459, 5.6642)
  line L440 (-37.7459, 5.6642) -> (-37.8729, 5.9182)
  line L441 (-37.8729, 5.9182) -> (-38.1269, 5.9182)
  line L442 (-38.1269, 5.9182) -> (-38.2539, 5.6642)
  line L443 (-38.2539, 5.6642) -> (-38.2539, 0.9906)
  line L444 (-38.2539, 0.9906) -> (-39.7459, 0.9906)
  line L445 (-39.7459, 0.9906) -> (-39.7459, 5.6642)
  line L446 (-39.7459, 5.6642) -> (-39.8729, 5.9182)
  line L447 (-39.8729, 5.9182) -> (-40.1269, 5.9182)
  line L448 (-40.1269, 5.9182) -> (-40.2539, 5.6642)
  line L449 (-40.2539, 5.6642) -> (-40.2539, 0.9906)
  line L450 (-40.2539, 0.9906) -> (-41.7459, 0.9906)
  line L451 (-41.7459, 0.9906) -> (-41.7459, 5.6642)
  line L452 (-41.7459, 5.6642) -> (-41.8729, 5.9182)
  line L453 (-41.8729, 5.9182) -> (-42.1269, 5.9182)
  line L454 (-42.1269, 5.9182) -> (-42.2539, 5.6642)
  line L455 (-42.2539, 5.6642) -> (-42.2539, 0.9906)
  line L456 (-42.2539, 0.9906) -> (-43.7459, 0.9906)
  line L457 (-43.7459, 0.9906) -> (-43.7459, 5.6642)
  line L458 (-43.7459, 5.6642) -> (-43.8729, 5.9182)
  line L459 (-43.8729, 5.9182) -> (-44.1269, 5.9182)
  line L460 (-44.1269, 5.9182) -> (-44.2539, 5.6642)
  line L461 (-44.2539, 5.6642) -> (-44.2539, 0.9906)
  line L462 (-44.2539, 0.9906) -> (-45.7459, 0.9906)
  line L463 (-45.7459, 0.9906) -> (-45.7459, 5.6642)
  line L464 (-45.7459, 5.6642) -> (-45.8729, 5.9182)
  line L465 (-45.8729, 5.9182) -> (-46.1269, 5.9182)
  line L466 (-46.1269, 5.9182) -> (-46.2539, 5.6642)
  line L467 (-46.2539, 5.6642) -> (-46.2539, 0.9906)
  line L468 (-46.2539, 0.9906) -> (-47.7459, 0.9906)
  line L469 (-47.7459, 0.9906) -> (-47.7459, 5.6642)
  line L470 (-47.7459, 5.6642) -> (-47.8729, 5.9182)
  line L471 (-47.8729, 5.9182) -> (-48.1269, 5.9182)
  line L472 (-48.1269, 5.9182) -> (-48.2539, 5.6642)
  line L473 (-48.2539, 5.6642) -> (-48.2539, 0.9906)
  line L474 (-48.2539, 0.9906) -> (-49.7459, 0.9906)
  line L475 (-49.7459, 0.9906) -> (-49.7459, 5.6642)
  line L476 (-49.7459, 5.6642) -> (-49.8729, 5.9182)
  line L477 (-49.8729, 5.9182) -> (-50.1269, 5.9182)
  line L478 (-50.1269, 5.9182) -> (-50.2539, 5.6642)
  line L479 (-50.2539, 5.6642) -> (-50.2539, 0.9906)
  line L480 (-50.2539, 0.9906) -> (-51.7459, 0.9906)
  line L481 (-51.7459, 0.9906) -> (-51.7459, 5.6642)
  line L482 (-51.7459, 5.6642) -> (-51.8729, 5.9182)
  line L483 (-51.8729, 5.9182) -> (-52.1269, 5.9182)
  line L484 (-52.1269, 5.9182) -> (-52.2539, 5.6642)
  line L485 (-52.2539, 5.6642) -> (-52.2539, 0.9906)
  line L486 (-52.2539, 0.9906) -> (-53.7459, 0.9906)
  line L487 (-53.7459, 0.9906) -> (-53.7459, 5.6642)
  line L488 (-53.7459, 5.6642) -> (-53.8729, 5.9182)
  line L489 (-53.8729, 5.9182) -> (-54.1269, 5.9182)
  line L490 (-54.1269, 5.9182) -> (-54.2539, 5.6642)
  line L491 (-54.2539, 5.6642) -> (-54.2539, 0.9906)
  line L492 (-54.2539, 0.9906) -> (-55.7459, 0.9906)
  line L493 (-55.7459, 0.9906) -> (-55.7459, 5.6642)
  line L494 (-55.7459, 5.6642) -> (-55.8729, 5.9182)
  line L495 (-55.8729, 5.9182) -> (-56.1269, 5.9182)
  line L496 (-56.1269, 5.9182) -> (-56.2539, 5.6642)
  line L497 (-56.2539, 5.6642) -> (-56.2539, 0.9906)
  line L498 (-56.2539, 0.9906) -> (-57.7459, 0.9906)
  line L499 (-57.7459, 0.9906) -> (-57.7459, 5.6642)
  line L500 (-57.7459, 5.6642) -> (-57.8729, 5.9182)
  line L501 (-57.8729, 5.9182) -> (-58.1269, 5.9182)
  line L502 (-58.1269, 5.9182) -> (-58.2539, 5.6642)
  line L503 (-58.2539, 5.6642) -> (-58.2539, 0.9906)
  line L504 (-58.2539, 0.9906) -> (-59.7459, 0.9906)
  line L505 (-59.7459, 0.9906) -> (-59.7459, 5.6642)
  line L506 (-59.7459, 5.6642) -> (-59.8729, 5.9182)
  line L507 (-59.8729, 5.9182) -> (-60.1269, 5.9182)
  line L508 (-60.1269, 5.9182) -> (-60.2539, 5.6642)
  line L509 (-60.2539, 5.6642) -> (-60.2539, 0.9906)
  line L510 (-60.2539, 0.9906) -> (-61.7459, 0.9906)
  line L511 (-61.7459, 0.9906) -> (-61.7459, 5.6642)
  line L512 (-61.7459, 5.6642) -> (-61.8729, 5.9182)
  line L513 (-61.8729, 5.9182) -> (-62.1269, 5.9182)
  line L514 (-62.1269, 5.9182) -> (-62.2539, 5.6642)
  line L515 (-62.2539, 5.6642) -> (-62.2539, 0.9906)
  line L516 (-62.2539, 0.9906) -> (-63.7459, 0.9906)
  line L517 (-63.7459, 0.9906) -> (-63.7459, 5.6642)
  line L518 (-63.7459, 5.6642) -> (-63.8729, 5.9182)
  line L519 (-63.8729, 5.9182) -> (-64.1269, 5.9182)
  line L520 (-64.1269, 5.9182) -> (-64.2539, 5.6642)
  line L521 (-64.2539, 5.6642) -> (-64.2539, 0.9906)
  line L522 (-64.2539, 0.9906) -> (-65.7459, 0.9906)
  line L523 (-65.7459, 0.9906) -> (-65.7459, 5.6642)
  line L524 (-65.7459, 5.6642) -> (-65.8729, 5.9182)
  line L525 (-65.8729, 5.9182) -> (-66.1269, 5.9182)
  line L526 (-66.1269, 5.9182) -> (-66.2539, 5.6642)
  line L527 (-66.2539, 5.6642) -> (-66.2539, 0.9906)
  line L528 (-66.2539, 0.9906) -> (-67.7459, 0.9906)
  line L529 (-67.7459, 0.9906) -> (-67.7459, 5.6642)
  line L530 (-67.7459, 5.6642) -> (-67.8729, 5.9182)
  line L531 (-67.8729, 5.9182) -> (-68.1269, 5.9182)
  line L532 (-68.1269, 5.9182) -> (-68.2539, 5.6642)
  line L533 (-68.2539, 5.6642) -> (-68.2539, 0.9906)
  line L534 (-68.2539, 0.9906) -> (-69.7459, 0.9906)
  line L535 (-69.7459, 0.9906) -> (-69.7459, 5.6642)
  line L536 (-69.7459, 5.6642) -> (-69.8729, 5.9182)
  line L537 (-69.8729, 5.9182) -> (-70.1269, 5.9182)
  line L538 (-70.1269, 5.9182) -> (-70.2539, 5.6642)
  line L539 (-70.2539, 5.6642) -> (-70.2539, 0.9906)
  line L540 (-70.2539, 0.9906) -> (-71.7459, 0.9906)
  line L541 (-71.7459, 0.9906) -> (-71.7459, 5.6642)
  line L542 (-71.7459, 5.6642) -> (-71.8729, 5.9182)
  line L543 (-71.8729, 5.9182) -> (-72.1269, 5.9182)
  line L544 (-72.1269, 5.9182) -> (-72.2539, 5.6642)
  line L545 (-72.2539, 5.6642) -> (-72.2539, 0.9906)
  line L546 (-72.2539, 0.9906) -> (-73.7459, 0.9906)
  line L547 (-73.7459, 0.9906) -> (-73.7459, 5.6642)
  line L548 (-73.7459, 5.6642) -> (-73.8729, 5.9182)
  line L549 (-73.8729, 5.9182) -> (-74.1269, 5.9182)
  line L550 (-74.1269, 5.9182) -> (-74.2539, 5.6642)
  line L551 (-74.2539, 5.6642) -> (-74.2539, 0.9906)
  line L552 (-74.2539, 0.9906) -> (-75.7458, 0.9906)
  line L553 (-75.7458, 0.9906) -> (-75.7458, 5.6642)
  line L554 (-75.7458, 5.6642) -> (-75.8728, 5.9182)
  line L555 (-75.8728, 5.9182) -> (-76.1268, 5.9182)
  line L556 (-76.1268, 5.9182) -> (-76.2538, 5.6642)
  line L557 (-76.2538, 5.6642) -> (-76.2538, 0.9906)
  line L558 (-76.2538, 0.9906) -> (-77.7458, 0.9906)
  line L559 (-77.7458, 0.9906) -> (-77.7458, 5.6642)
  line L560 (-77.7458, 5.6642) -> (-77.8728, 5.9182)
  line L561 (-77.8728, 5.9182) -> (-78.1268, 5.9182)
  line L562 (-78.1268, 5.9182) -> (-78.2538, 5.6642)
  line L563 (-78.2538, 5.6642) -> (-78.2538, 0.9906)
  line L564 (-78.2538, 0.9906) -> (-79.7458, 0.9906)
  line L565 (-79.7458, 0.9906) -> (-79.7458, 5.6642)
  line L566 (-79.7458, 5.6642) -> (-79.8728, 5.9182)
  line L567 (-79.8728, 5.9182) -> (-80.1268, 5.9182)
  line L568 (-80.1268, 5.9182) -> (-80.2538, 5.6642)
  line L569 (-80.2538, 5.6642) -> (-80.2538, 0.9906)
  line L570 (-80.2538, 0.9906) -> (-81.7458, 0.9906)
  line L571 (-81.7458, 0.9906) -> (-81.7458, 5.6642)
  line L572 (-81.7458, 5.6642) -> (-81.8728, 5.9182)
  line L573 (-81.8728, 5.9182) -> (-82.1268, 5.9182)
  line L574 (-82.1268, 5.9182) -> (-82.2538, 5.6642)
  line L575 (-82.2538, 5.6642) -> (-82.2538, 0.9906)
  line L576 (-82.2538, 0.9906) -> (-83.7458, 0.9906)
  line L577 (-83.7458, 0.9906) -> (-83.7458, 5.6642)
  line L578 (-83.7458, 5.6642) -> (-83.8728, 5.9182)
  line L579 (-83.8728, 5.9182) -> (-84.1268, 5.9182)
  line L580 (-84.1268, 5.9182) -> (-84.2538, 5.6642)
  line L581 (-84.2538, 5.6642) -> (-84.2538, 0.9906)
  line L582 (-84.2538, 0.9906) -> (-85.7458, 0.9906)
  line L583 (-85.7458, 0.9906) -> (-85.7458, 5.6642)
  line L584 (-85.7458, 5.6642) -> (-85.8728, 5.9182)
  line L585 (-85.8728, 5.9182) -> (-86.1268, 5.9182)
  line L586 (-86.1268, 5.9182) -> (-86.2538, 5.6642)
  line L587 (-86.2538, 5.6642) -> (-86.2538, 0.9906)
  line L588 (-86.2538, 0.9906) -> (-87.7458, 0.9906)
  line L589 (-87.7458, 0.9906) -> (-87.7458, 5.6642)
  line L590 (-87.7458, 5.6642) -> (-87.8728, 5.9182)
  line L591 (-87.8728, 5.9182) -> (-88.1268, 5.9182)
  line L592 (-88.1268, 5.9182) -> (-88.2538, 5.6642)
  line L593 (-88.2538, 5.6642) -> (-88.2538, 0.9906)
  line L594 (-88.2538, 0.9906) -> (-89.7458, 0.9906)
  line L595 (-89.7458, 0.9906) -> (-89.7458, 5.6642)
  line L596 (-89.7458, 5.6642) -> (-89.8728, 5.9182)
  line L597 (-89.8728, 5.9182) -> (-90.1268, 5.9182)
  line L598 (-90.1268, 5.9182) -> (-90.2538, 5.6642)
  line L599 (-90.2538, 5.6642) -> (-90.2538, 0.9906)
  line L600 (-90.2538, 0.9906) -> (-91.7458, 0.9906)
  line L601 (-91.7458, 0.9906) -> (-91.7458, 5.6642)
  line L602 (-91.7458, 5.6642) -> (-91.8728, 5.9182)
  line L603 (-91.8728, 5.9182) -> (-92.1268, 5.9182)
  line L604 (-92.1268, 5.9182) -> (-92.2538, 5.6642)
  line L605 (-92.2538, 5.6642) -> (-92.2538, 0.9906)
  line L606 (-92.2538, 0.9906) -> (-93.7458, 0.9906)
  line L607 (-93.7458, 0.9906) -> (-93.7458, 5.6642)
  line L608 (-93.7458, 5.6642) -> (-93.8728, 5.9182)
  line L609 (-93.8728, 5.9182) -> (-94.1268, 5.9182)
  line L610 (-94.1268, 5.9182) -> (-94.2538, 5.6642)
  line L611 (-94.2538, 5.6642) -> (-94.2538, 0.9906)
  line L612 (-94.2538, 0.9906) -> (-95.7458, 0.9906)
  line L613 (-95.7458, 0.9906) -> (-95.7458, 5.6642)
  line L614 (-95.7458, 5.6642) -> (-95.8728, 5.9182)
  line L615 (-95.8728, 5.9182) -> (-96.1268, 5.9182)
  line L616 (-96.1268, 5.9182) -> (-96.2538, 5.6642)
  line L617 (-96.2538, 5.6642) -> (-96.2538, 0.9906)
  line L618 (-96.2538, 0.9906) -> (-97.7458, 0.9906)
  line L619 (-97.7458, 0.9906) -> (-97.7458, 5.6642)
  line L620 (-97.7458, 5.6642) -> (-97.8728, 5.9182)
  line L621 (-97.8728, 5.9182) -> (-98.1268, 5.9182)
  line L622 (-98.1268, 5.9182) -> (-98.2538, 5.6642)
  line L623 (-98.2538, 5.6642) -> (-98.2538, 0.9906)
  line L624 (-98.2538, 0.9906) -> (-99.7458, 0.9906)
  line L625 (-99.7458, 0.9906) -> (-99.7458, 5.6642)
  line L626 (-99.7458, 5.6642) -> (-99.8728, 5.9182)
  line L627 (-99.8728, 5.9182) -> (-100.1268, 5.9182)
  line L628 (-100.1268, 5.9182) -> (-100.2538, 5.6642)
  line L629 (-100.2538, 5.6642) -> (-100.2538, 0.9906)
  line L630 (-100.2538, 0.9906) -> (-100.4603, 0.9906)
  line L631 (-100.4603, 0.9906) -> (-100.4603, 0.762)
  constraints: 1264 end point
extrude "Extrusion2" cut sketch "Sketch_1" along normal mid plane 15.24
ref_plane "0_XY" through (0, 0, 0) normal (0, 1, 0) x (1, 0, 0)
ref_plane "0_YZ" through (0, 0, 0) normal (1, 0, 0) x (0, 0, -1)
ref_plane "0_ZX" through (0, 0, 0) normal (0, 0, -1) x (0, 1, 0)
body "Solid1"
